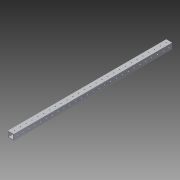
# Autodesk Inventor part: chassis front back rail
Saved by Autodesk Inventor 2014 SP1 (Build 180222100, 222)
## iProperties
Created: 2014-01-04
Part Number: chassis front back rail
Material: Aluminum 6061
Document SubType Name: Modeling
Designer: Arpan
Density: 2.71 g/cm^3
Appearance: Aluminum - Flat
Author: Arpan
Autodesk Inventor part; units mm, degrees
ref_plane "YZ Plane" through (0, 0, 0) normal (1, 0, 0) x (0, 1, 0)
ref_plane "XZ Plane" through (0, 0, 0) normal (0, 1, 0) x (-1, 0, 0)
ref_plane "XY Plane" through (0, 0, 0) normal (0, 0, 1) x (1, 0, 0)
sketch "Sketch1" plane through (0, 0, 0) normal (0, 0, 1) x (1, 0, 0)
  line L0 (0, 0) -> (-25.4, 0)
  line L1 (-25.4, 0) -> (-25.4, 25.4)
  line L2 (-25.4, 25.4) -> (0, 25.4)
  line L3 (0, 25.4) -> (0, 0)
  line L4 (-3.175, 22.225) -> (-22.225, 22.225)
  line L5 (-22.225, 22.225) -> (-22.225, 3.175)
  line L6 (-22.225, 3.175) -> (-3.175, 3.175)
  line L7 (-3.175, 3.175) -> (-3.175, 22.225)
  dimension "d0" = 25.4
  dimension "d1" = 25.4
  dimension "d2" = 3.175
  constraints: 16 end point, 4 parallel, 2 perpendicular, 1 horizontal, 3 other
  measures "d0" distance of L0.end L1.end
  measures "d1" distance of L1.end L2.end
  measures "d2" distance between parallel lines of L2 L4
extrude "Extrusion1" add sketch "Sketch1" along normal blind 688.975
sketch "Sketch3" plane through (-25.4, 25.4, 0) normal (0, 1, 0) x (1, 0, 0)
  line L0 (0, 0) -> (25.4, 0) projected
  line L1 (25.4, 0) -> (25.4, -688.975) projected
  line L2 (12.7, 0) -> (12.7, -12.7)
  circle A0 centre (12.7, -12.7) radius 2.0828
  dimension "d5" = 12.7
  dimension "d6" = 4.1656
  constraints: 2 end point, 1 centre point, 1 coincident, 1 midpoint, 1 parallel
  measures "d5" distance of L2.start L2.end
  measures "d6" diameter of A0
extrude "Extrusion2" cut sketch "Sketch3" against normal blind 25.4
sketch "Sketch2" plane through (-25.4, 0, 0) normal (-1, 0, 0) x (0, 0, 1)
  line L0 (0, 0) -> (0, 25.4) projected
  line L1 (0, 0) -> (688.975, 0) projected
  line L2 (688.975, 25.4) -> (688.975, 0) projected
  line L3 (0, 25.4) -> (688.975, 25.4) projected
  line L4 (0, 12.7) -> (12.7, 12.7)
  circle A0 centre (12.7, 12.7) radius 2.0828
  dimension "d12" = 12.7
  dimension "d13" = 4.1656
  constraints: 2 end point, 1 centre point, 1 coincident, 1 midpoint, 1 parallel
  measures "d12" distance of L4.start L4.end
  measures "d13" diameter of A0
pattern_linear "Rectangular Pattern1" count 27 spacing 25.4 along (0, 0, 1) of "Extrusion2"
extrude "Extrusion3" cut sketch "Sketch2" against normal blind 25.4 contours A0
pattern_linear "Rectangular Pattern2" count 27 spacing 25.4 along (0, 0, 1) of "Extrusion3"
body "Solid1"
